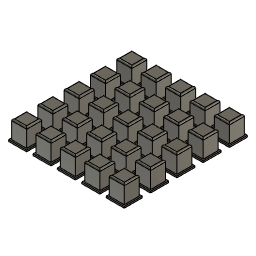
midi button with feet (Autodesk Fusion 360 design; units mm, degrees)
Autodesk Fusion 360 part; units mm, degrees
note: some values were not read from the file. Chosen so that the rebuilt part matches the saved one: which bodies a step acts on.
sketch "Sketch1" plane through (0, 0, 0) normal (0, 0, 1) x (1, 0, 0)
  line L0 (0, 0) -> (10, 0)
  line L1 (10, 0) -> (10, 10)
  line L2 (10, 10) -> (0, 10)
  line L3 (0, 10) -> (0, 0)
  line L4 (0, 10) -> (-1, 10)
  line L5 (-1, 10) -> (-1, 11)
  line L6 (-1, 11) -> (0, 11)
  line L7 (0, 11) -> (0, 10)
  line L8 (-1, 11) -> (11, 11)
  line L9 (11, 11) -> (11, -1)
  line L10 (11, -1) -> (-1, -1)
  line L11 (-1, -1) -> (-1, 11)
  dimension "d1" = 10
  dimension "d2" = 10
  dimension "d7" = 1
  dimension "d8" = 1
  dimension "d9" = 12
  dimension "d10" = 12
  constraint horizontal L0
  constraint vertical L1
  constraint horizontal L2
  constraint vertical L3
  constraint coincident L0.start L3.end
  constraint horizontal L4
  constraint vertical L5
  constraint horizontal L6
  constraint vertical L7
  constraint horizontal L8
  constraint vertical L9
  constraint horizontal L10
  constraint vertical L11
  measures "d1" distance of L0.start L0.end
  measures "d2" distance of L0.start L2.end
  measures "d7" distance of L2.end L4.end
  measures "d8" distance of L2.end L6.end
  measures "d9" distance of L5.end L8.end
  measures "d10" distance of L5.end L10.end
extrude "Extrude1" add sketch "Sketch1" along normal blind 13 contours L0 L1 L2 L3 makes body 1
shell "Shell1" thickness 1 removed faces 0 bodies 1
fillet "Fillet1" radius 1 4 edges at (5, 0, 13) (0, 5, 13) (5, 10, 13) (10, 5, 13) on bodies 1
extrude "Extrude2" add sketch "Sketch1" along normal blind 1 bodies 1
pattern_linear "R-Pattern1" count 1 spacing 0 along (0, 0, 1) count 5 spacing 17.5 along (0, -1, 0) of bodies 1 makes body 2 at (3, -10.5, 0) makes body 3 at (3, -28, 0) makes body 4 at (3, -49.5, 0) makes body 5 at (3, -67, 0)
pattern_linear "R-Pattern2" count 1 spacing 0 along (0, 1, 0) count 5 spacing 16.25 along (1, 0, 0) of bodies 1 4 3 2 5 makes body 6 at (23.25, 3, 0) makes body 7 at (39.5, 3, 0) makes body 8 at (55.75, 3, 0) makes body 9 at (72, 3, 0) makes body 10 at (23.25, -32, 0) makes body 11 at (35.5, -28, 0) makes body 12 at (51.75, -28, 0) makes body 13 at (68, -28, 0) makes body 14 at (23.25, -14.5, 0) makes body 15 at (35.5, -10.5, 0) makes body 16 at (51.75, -10.5, 0) makes body 17 at (68, -10.5, 0) makes body 18 at (23.25, -49.5, 0) makes body 19 at (35.5, -45.5, 0) makes body 20 at (51.75, -45.5, 0) makes body 21 at (68, -49.5, 0) makes body 22 at (23.25, -67, 0) makes body 23 at (35.5, -63, 0) makes body 24 at (51.75, -63, 0) makes body 25 at (68, -67, 0)
